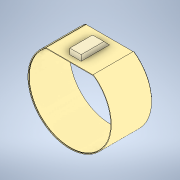
# Autodesk Inventor part: Large_Ring
Saved by Autodesk Inventor 2021 (Build 250183000, 183)
## iProperties
Created: 2020-05-28
Part Number: Large_Ring
Material: Generic
Document SubType Name: Modeling
Designer: aydan
Density: 1 g/cm^3
Appearance: Gold - Metal
Author: aydan
Autodesk Inventor part; units mm, degrees
ref_plane "YZ Plane" through (0, 0, 0) normal (1, 0, 0) x (0, 1, 0)
sketch "Sketch1" plane through (0, 0, 0) normal (0, 0, 1) x (1, 0, 0)
  circle A0 centre (0, 0) radius 17.25
  circle A1 centre (0, 0) radius 17.375
  dimension "d0" = 34.5
  dimension "d1" = 34.75
  constraints: 2 centre point, 2 coincident
  measures "d0" diameter of A0
  measures "d1" diameter of A1
extrude "Extrusion1" add sketch "Sketch1" along normal mid plane 17
sketch "Sketch2" plane through (0, 0, 0) normal (0, 0, 1) x (1, 0, 0)
  circle A0 centre (0, 0) radius 17.375
  circle A1 centre (0, 0) radius 17.625
  dimension "d4" = 34.75
  dimension "d5" = 0.25
  constraints: 2 centre point, 1 coincident
  measures "d4" diameter of A0
  measures "d5" radial gap between concentric circles of A0 A1
extrude "Extrusion2" add sketch "Sketch2" along normal blind 8.75 and the other way blind 8.25
ref_plane "Work Plane1" through (0, 17.625, 0) normal (0, 1, 0) x (-1, 0, 0)
sketch "Sketch3" plane through (0, 17.625, 0) normal (0, 1, 0) x (-1, 0, 0)
  line L0 (10, 0) -> (10, -8.5)
  line L1 (10, -8.5) -> (0, -8.5)
  line L2 (-10, 0) -> (-10, 9.4902)
  line L3 (-10, 9.4902) -> (-0.099, 9.4902)
  line L4 (10, -8.5) -> (-10, -8.5)
  line L5 (-10, -8.5) -> (-10, 9.4902)
  line L6 (-10, 9.4902) -> (10, 9.4902)
  line L7 (10, 9.4902) -> (10, -8.5)
  point P0 (0, 0)
  point P1 (-0.099, 9.4902)
  dimension "d10" = 10
  dimension "d11" = 10
  constraints: 16 end point, 2 parallel, 1 horizontal, 1 perpendicular
  measures "d10" distance of point (0, 0) L0.start
  measures "d11" distance of point (0, 0) L2.start
extrude "Extrusion3" cut sketch "Sketch3" against normal blind 8.75
ref_plane "Work Plane2" through (0, 14.1, 0) normal (0, 1, 0) x (-1, 0, 0)
sketch "Sketch4" plane through (0, 14.1, 0) normal (0, 1, 0) x (-1, 0, 0)
  line L0 (-10, -8.25) -> (-10, 8.75) projected
  line L1 (10, -8.25) -> (-10, -8.25)
  line L2 (-10, -8.25) -> (-10, 8.75)
  line L3 (-10, 8.75) -> (10, 8.75)
  line L4 (10, 8.75) -> (10, -8.25)
  point P0 (0, 0)
  constraints: 8 end point, 2 parallel, 1 horizontal, 1 perpendicular
extrude "Extrusion4" add sketch "Sketch4" along normal blind 0.25
sketch "Sketch5" plane through (0, 14.35, 0) normal (0, 1, 0) x (1, 0, 0)
  line L0 (-2.4, 5.75) -> (2.4, 5.75)
  line L1 (2.4, 5.75) -> (2.4, -6.25)
  line L2 (2.4, -6.25) -> (-2.4, -6.25)
  line L3 (-2.4, -6.25) -> (-2.4, 5.75)
  line L4 (10, 8.25) -> (-10, 8.25) projected
  line L5 (10, 8.25) -> (10, -8.75) projected
  point P0 (0, 0)
  dimension "d17" = 4.8
  dimension "d18" = 12
  dimension "d19" = 2.5
  dimension "d20" = 7.6
  constraints: 8 end point, 2 parallel, 1 horizontal, 1 perpendicular
  measures "d17" distance of L1.end L2.end
  measures "d18" distance of L0.end L1.end
  measures "d19" distance between parallel lines of L4 L0
  measures "d20" distance between parallel lines of L5 L1
extrude "Extrusion5" add sketch "Sketch5" along normal blind 2.4
sketch "Sketch6" plane through (2.4, 14.35, 6.25) normal (1, 0, 0) x (0, 0, -1)
  line L0 (12, 0) -> (12, 2.4) projected
  line L1 (12, 0) -> (9.6, 2.4)
  line L2 (12, 2.4) -> (0, 2.4) projected
  line L3 (12, 0) -> (15.3941, 0) construction
  line L4 (9.6, 2.4) -> (12, 2.4)
  line L5 (12, 2.4) -> (12, 0)
  point P0 (6.25, -14.35)
  dimension "d23" = 135
  constraints: 8 end point, 2 collinear, 1 equal length, 1 horizontal, 1 point on line
  measures "d23" angle of L3 L1
extrude "Extrusion6" cut sketch "Sketch6" against normal blind 4.8
body "Solid1"
